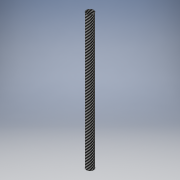
# Autodesk Inventor part: feet type 3 part 2 2k8 length
Saved by Autodesk Inventor 2018 (Build 220112000, 112)
## iProperties
Created: 2018-12-06
Part Number: feet type 3 part 2 2k8 length
Material: CFRP
Document SubType Name: Modeling
Designer: freyja
Density: 1.43 g/cm^3
Appearance: Carbon Fiber
Author: freyja
Autodesk Inventor part; units mm, degrees
ref_plane "YZ Plane" through (0, 0, 0) normal (1, 0, 0) x (0, 1, 0)
ref_plane "XZ Plane" through (0, 0, 0) normal (0, 1, 0) x (-1, 0, 0)
ref_plane "XY Plane" through (0, 0, 0) normal (0, 0, 1) x (1, 0, 0)
sketch "Sketch1" plane through (0, 0, 0) normal (0, 1, 0) x (-1, 0, 0)
  circle A0 centre (0, 0) radius 5.334
  circle A1 centre (0, 0) radius 4.953
  dimension "d0" = 10.668
  dimension "d1" = 9.906
  constraints: 2 centre point, 2 coincident
  measures "d0" diameter of A0
  measures "d1" diameter of A1
extrude "Extrusion1" add sketch "Sketch1" along normal blind 199.1194
body "Solid1"
